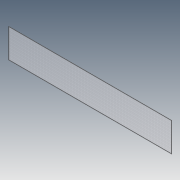
# Autodesk Inventor part: GE-12104
Saved by Autodesk Inventor 2012 (Build 160160000, 160)
## iProperties
Created: 2011-10-29
Part Number: GE-12104
Document SubType Name: Modeling
Designer: dfoster
Density: 1 g/cm^3
Description: Net, End Panel
Material: Default
Title: Net, End Panel
Author: dfoster
Autodesk Inventor part; units mm, degrees
ref_plane "YZ Plane" through (0, 0, 0) normal (1, 0, 0) x (0, 1, 0)
ref_plane "XZ Plane" through (0, 0, 0) normal (0, 1, 0) x (-1, 0, 0)
ref_plane "XY Plane" through (0, 0, 0) normal (0, 0, 1) x (1, 0, 0)
sketch "Sketch1" plane through (0, 0, 0) normal (0, 0, 1) x (1, 0, 0)
  line L0 (0, 0) -> (6791.96, 0)
  line L1 (6791.96, 0) -> (6791.96, 1219.2)
  line L2 (6791.96, 1219.2) -> (0, 1219.2)
  line L3 (0, 1219.2) -> (0, 0)
  line L4 (12.7, 1206.5) -> (6779.26, 1206.5)
  line L5 (6779.26, 1206.5) -> (6779.26, 12.7)
  line L6 (6779.26, 12.7) -> (12.7, 12.7)
  line L7 (12.7, 12.7) -> (12.7, 1206.5)
  dimension "d0" = 6791.96
  dimension "d1" = 1219.2
  dimension "d4" = 12.7
  constraints: 16 end point, 4 parallel, 2 perpendicular, 1 horizontal, 3 other
  measures "d0" distance of L1.end L2.end
  measures "d1" distance of L2.end L0.start
  measures "d4" distance between parallel lines of L4 L2
extrude "Extrusion1" add sketch "Sketch1" along normal mid plane 6.35 contours L3 L2 L1 L0 | L4 L5 L6 L7
extrude "Extrusion2" add sketch "Sketch1" along normal mid plane 12.7
body "Solid1"
